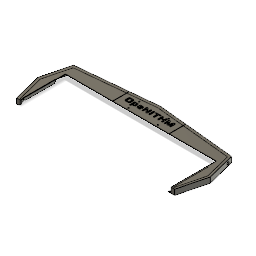
Frame v10 (Autodesk Fusion 360 design; units mm, degrees)
Autodesk Fusion 360 part; units mm, degrees
sketch "Sketch1" plane through (0, 0, 0) normal (0, 1, 0) x (1, 0, 0)
  line L0 (240, 0) -> (240, -144)
  line L1 (240, -144) -> (252, -144)
  line L2 (252, -144) -> (275, -53)
  line L3 (275, -53) -> (252, 38)
  line L4 (252, 38) -> (0, 63)
  line L5 (0, 63) -> (0, 0)
  line L6 (0, 0) -> (240, 0)
  dimension "d1" = 63
  dimension "d2" = 12
  dimension "d4" = 240
  dimension "d5" = 144
  dimension "d6" = 35
  dimension "d7" = 12
  dimension "d8" = 182
  measures "d1" distance of L5.end
extrude "Extrude1" add sketch "Sketch1" along normal blind 17.5 makes body 1
sketch "Sketch2" plane through (0, 0, 0) normal (0, -1, 0) x (1, 0, 0)
  line L0 (240, 0) -> (0, 0)
  line L1 (0, 0) -> (0, -63)
  line L2 (0, -63) -> (252, -38)
  line L3 (252, -38) -> (275, 53)
  line L4 (275, 53) -> (252, 144)
  line L5 (252, 144) -> (240, 144)
  line L6 (240, 144) -> (240, 0)
  line L7 (0, -55) -> (245.8682, -30.6083)
  line L8 (245.8682, -30.6083) -> (267, 53)
  line L9 (0, -55) -> (0, 0)
  line L10 (240, 0) -> (0, 0)
  line L11 (240, 0) -> (240, 139)
  line L12 (275, 53) -> (267, 53) construction
  line L13 (0, -63) -> (0, -55) construction
  line L14 (240, 139) -> (245.2637, 139)
  line L15 (245.2637, 139) -> (267, 53)
  dimension "d11" = 5
  dimension "d12" = 8
  dimension "d13" = 8
extrude "Extrude2" cut sketch "Sketch2" against normal blind 16 contours L0 L1 L6 L7 L8 L9 L10 L11 L14 L15 bodies 1
sketch "Sketch3" plane through (0, 0, 0) normal (-1, 0, 0) x (0, 0, 1)
  line L0 (-55, 0) -> (-55, 16)
  line L1 (-55, 16) -> (0, 16)
  line L2 (0, 16) -> (0, 17.5)
  line L3 (0, 17.5) -> (-63, 17.5)
  line L4 (-63, 17.5) -> (-63, 0)
  line L5 (-63, 0) -> (-55, 0)
  circle A0 centre (-22.6083, 8) radius 4
  line L6 (53, 0) -> (-30.6083, 0)
  line L7 (-30.6083, 0) -> (-30.6083, 16)
  dimension "d16" = 8
  dimension "d17" = 8
  dimension "d18" = 8
  measures "d16" diameter of A0
  measures "d17" distance of L6
  measures "d18" distance of L7
extrude "Extrude3" cut sketch "Sketch3" against normal through all contours A0 bodies 1
sketch "Sketch4" plane through (0, 0, 0) normal (0, 0, 1) x (1, 0, 0)
  line L0 (0, 16) -> (240, 16)
  line L1 (240, 16) -> (240, 17.5)
  line L2 (240, 17.5) -> (0, 17.5)
  line L3 (0, 17.5) -> (0, 16)
  line L4 (-8, 4) -> (8, 4)
  arc A0 (8, 4) -> (8, 12) centre (8, 8) ccw
  line L5 (8, 12) -> (-8, 12)
  arc A1 (-8, 12) -> (-8, 4) centre (-8, 8) ccw
  line L6 (-8, 8) -> (8, 8) construction
  line L7 (0, 0) -> (0, 17.5)
  line L8 (245.8682, 0) -> (0, 0)
  dimension "d20" = 8
  dimension "d21" = 12
  dimension "d22" = 8
  measures "d20" distance of L4 L5
  measures "d22" distance of L6 L8
extrude "Extrude4" cut sketch "Sketch4" against normal through all contours L4 A0 L5 L7 bodies 1
mirror "Mirror1" about plane through (0, 0, 0) normal (1, 0, 0) of "Extrude1", "Extrude2", "Extrude3", "Extrude4" makes body 2
combine "Combine1" operation add target body 1 tool bodies 2
sketch "Sketch5" plane through (0, 0, 144) normal (0, 0, 1) x (1, 0, 0)
  line L0 (240, 0) -> (252, 0)
  line L1 (252, 0) -> (252, 17.5)
  line L2 (252, 17.5) -> (240, 17.5)
  line L3 (240, 17.5) -> (240, 0)
  line L4 (245.8682, 0) -> (0, 0)
  line L5 (240, 0) -> (230, 0)
  line L6 (240, 3.7) -> (230, 0)
  line L7 (240, 0) -> (240, 3.7)
  dimension "d25" = 10
  dimension "d26" = 3.7
  measures "d26" distance of L4.end
extrude "Extrude5" add sketch "Sketch5" against normal blind 5 contours L3 L4 L5 L6 L7 bodies 1
sketch "Sketch6" plane through (0, 0, 144) normal (0, 0, 1) x (1, 0, 0)
  line L0 (-252, 0) -> (-240, 0)
  line L1 (-240, 0) -> (-240, 17.5)
  line L2 (-240, 17.5) -> (-252, 17.5)
  line L3 (-252, 17.5) -> (-252, 0)
  line L4 (-240, 0) -> (-240, 3.7)
  line L5 (-250, 0) -> (-240, 3.7)
  line L6 (-240, 0) -> (-250, 0)
  dimension "d29" = 3.7
  dimension "d30" = 10
  measures "d29" distance of origin
extrude "Extrude6" cut sketch "Sketch6" against normal blind 5 contours L0 L1 L4 L5 L6 bodies 1
ref_plane "WorkPlane1" through (0, 22.5, 40.5) normal (0, 1, 0) x (0, 0, 1)
sketch "Sketch7" plane through (0, 22.5, 0) normal (0, 1, 0) x (-1, 0, 0)
  line L0 (0, -41.653) -> (0, -63) construction
  line L1 (73.6847, -25.1213) -> (73.6847, -34.9739)
  spline S0 degree 2 poles (73.6847, -34.9739) (73.6847, -37.7889) (70.166, -37.7889) knots 0 0 0 1 1 1
  line L2 (70.166, -37.7889) -> (61.7209, -37.7889)
  spline S1 degree 2 poles (61.7209, -37.7889) (58.2021, -37.7889) (58.2021, -34.9739) knots 0 0 0 1 1 1
  line L3 (58.2021, -34.9739) -> (58.2021, -25.1213)
  spline S2 degree 2 poles (58.2021, -25.1213) (58.2021, -22.3062) (61.7209, -22.3062) knots 0 0 0 1 1 1
  line L4 (61.7209, -22.3062) -> (70.166, -22.3062)
  spline S3 degree 2 poles (70.166, -22.3062) (73.6847, -22.3062) (73.6847, -25.1213) knots 0 0 0 1 1 1
  spline S4 degree 2 poles (70.4005, -25.0509) (70.4005, -24.3002) (69.4622, -24.3002) knots 0 0 0 1 1 1
  line L5 (69.4622, -24.3002) -> (62.4246, -24.3002)
  spline S5 degree 2 poles (62.4246, -24.3002) (61.4863, -24.3002) (61.4863, -25.0509) knots 0 0 0 1 1 1
  line L6 (61.4863, -25.0509) -> (61.4863, -35.0443)
  spline S6 degree 2 poles (61.4863, -35.0443) (61.4863, -35.7949) (62.4246, -35.7949) knots 0 0 0 1 1 1
  line L7 (62.4246, -35.7949) -> (69.4622, -35.7949)
  spline S7 degree 2 poles (69.4622, -35.7949) (70.4005, -35.7949) (70.4005, -35.0443) knots 0 0 0 1 1 1
  line L8 (70.4005, -35.0443) -> (70.4005, -25.0509)
  line L9 (52.8552, -17.3799) -> (52.8552, -33.5664)
  line L10 (52.8552, -33.5664) -> (43.7063, -33.5664)
  spline S8 degree 2 poles (43.7063, -33.5664) (40.4221, -33.5664) (40.4221, -30.939) knots 0 0 0 1 1 1
  line L11 (40.4221, -30.939) -> (40.4221, -24.9336)
  spline S9 degree 2 poles (40.4221, -24.9336) (40.4221, -22.3062) (43.7063, -22.3062) knots 0 0 0 1 1 1
  line L12 (43.7063, -22.3062) -> (49.8056, -22.3062)
  line L13 (49.8056, -22.3062) -> (49.8056, -17.3799)
  line L14 (49.8056, -17.3799) -> (52.8552, -17.3799)
  line L15 (49.8056, -24.0656) -> (44.2928, -24.0656)
  spline S10 degree 2 poles (44.2928, -24.0656) (43.4718, -24.0656) (43.4718, -24.7225) knots 0 0 0 1 1 1
  line L16 (43.4718, -24.7225) -> (43.4718, -31.1501)
  spline S11 degree 2 poles (43.4718, -31.1501) (43.4718, -31.8069) (44.2928, -31.8069) knots 0 0 0 1 1 1
  line L17 (44.2928, -31.8069) -> (49.8056, -31.8069)
  line L18 (49.8056, -31.8069) -> (49.8056, -24.0656)
  line L19 (35.319, -24.9336) -> (35.319, -30.939)
  spline S12 degree 2 poles (35.319, -30.939) (35.319, -33.5664) (32.0348, -33.5664) knots 0 0 0 1 1 1
  line L20 (32.0348, -33.5664) -> (26.6393, -33.5664)
  spline S13 degree 2 poles (26.6393, -33.5664) (23.3551, -33.5664) (23.3551, -30.939) knots 0 0 0 1 1 1
  line L21 (23.3551, -30.939) -> (23.3551, -27.3498)
  line L22 (23.3551, -27.3498) -> (32.2694, -27.3498)
  line L23 (32.2694, -27.3498) -> (32.2694, -24.7225)
  spline S14 degree 2 poles (32.2694, -24.7225) (32.2694, -24.0656) (31.4483, -24.0656) knots 0 0 0 1 1 1
  line L24 (31.4483, -24.0656) -> (23.8243, -24.0656)
  line L25 (23.8243, -24.0656) -> (23.8243, -22.3062)
  line L26 (23.8243, -22.3062) -> (32.0348, -22.3062)
  spline S15 degree 2 poles (32.0348, -22.3062) (35.319, -22.3062) (35.319, -24.9336) knots 0 0 0 1 1 1
  line L27 (32.2694, -29.1092) -> (26.4047, -29.1092)
  line L28 (26.4047, -29.1092) -> (26.4047, -31.1501)
  spline S16 degree 2 poles (26.4047, -31.1501) (26.4047, -31.807) (27.2258, -31.807) knots 0 0 0 1 1 1
  line L29 (27.2258, -31.807) -> (31.4483, -31.807)
  spline S17 degree 2 poles (31.4483, -31.807) (32.2694, -31.807) (32.2694, -31.1501) knots 0 0 0 1 1 1
  line L30 (32.2694, -31.1501) -> (32.2694, -29.1092)
  line L31 (18.0064, -22.3062) -> (18.0064, -37.7889)
  line L32 (18.0064, -37.7889) -> (14.253, -37.7889)
  line L33 (14.253, -37.7889) -> (5.5733, -26.3411)
  line L34 (5.5733, -26.3411) -> (5.5733, -37.7889)
  line L35 (5.5733, -37.7889) -> (2.2891, -37.7889)
  line L36 (2.2891, -37.7889) -> (2.2891, -22.3062)
  line L37 (2.2891, -22.3062) -> (6.0425, -22.3062)
  line L38 (6.0425, -22.3062) -> (14.7222, -33.754)
  line L39 (14.7222, -33.754) -> (14.7222, -22.3062)
  line L40 (14.7222, -22.3062) -> (18.0064, -22.3062)
  line L41 (-3.2868, -22.3062) -> (-3.2868, -37.7889)
  line L42 (-3.2868, -37.7889) -> (-6.571, -37.7889)
  line L43 (-6.571, -37.7889) -> (-6.571, -22.3062)
  line L44 (-6.571, -22.3062) -> (-3.2868, -22.3062)
  line L45 (-10.9448, -35.7949) -> (-10.9448, -37.7889)
  line L46 (-10.9448, -37.7889) -> (-27.3658, -37.7889)
  line L47 (-27.3658, -37.7889) -> (-27.3658, -35.7949)
  line L48 (-27.3658, -35.7949) -> (-20.7974, -35.7949)
  line L49 (-20.7974, -35.7949) -> (-20.7974, -22.3062)
  line L50 (-20.7974, -22.3062) -> (-17.5132, -22.3062)
  line L51 (-17.5132, -22.3062) -> (-17.5132, -35.7949)
  line L52 (-17.5132, -35.7949) -> (-10.9448, -35.7949)
  line L53 (-31.7615, -22.3062) -> (-31.7615, -37.7889)
  line L54 (-31.7615, -37.7889) -> (-35.0457, -37.7889)
  line L55 (-35.0457, -37.7889) -> (-35.0457, -31.5724)
  line L56 (-35.0457, -31.5724) -> (-43.96, -31.5724)
  line L57 (-43.96, -31.5724) -> (-43.96, -37.7889)
  line L58 (-43.96, -37.7889) -> (-47.2442, -37.7889)
  line L59 (-47.2442, -37.7889) -> (-47.2442, -22.3062)
  line L60 (-47.2442, -22.3062) -> (-43.96, -22.3062)
  line L61 (-43.96, -22.3062) -> (-43.96, -29.5784)
  line L62 (-43.96, -29.5784) -> (-35.0457, -29.5784)
  line L63 (-35.0457, -29.5784) -> (-35.0457, -22.3062)
  line L64 (-35.0457, -22.3062) -> (-31.7615, -22.3062)
  line L65 (-52.8256, -22.3062) -> (-52.8256, -37.7889)
  line L66 (-52.8256, -37.7889) -> (-57.0482, -37.7889)
  line L67 (-57.0482, -37.7889) -> (-62.9128, -25.4966)
  line L68 (-62.9128, -25.4966) -> (-68.7775, -37.7889)
  line L69 (-68.7775, -37.7889) -> (-73.0001, -37.7889)
  line L70 (-73.0001, -37.7889) -> (-73.0001, -22.3062)
  line L71 (-73.0001, -22.3062) -> (-69.7158, -22.3062)
  line L72 (-69.7158, -22.3062) -> (-69.7158, -33.1206)
  line L73 (-69.7158, -33.1206) -> (-64.555, -22.3062)
  line L74 (-64.555, -22.3062) -> (-61.2708, -22.3062)
  line L75 (-61.2708, -22.3062) -> (-56.1099, -33.1206)
  line L76 (-56.1099, -33.1206) -> (-56.1099, -22.3062)
  line L77 (-56.1099, -22.3062) -> (-52.8256, -22.3062)
split_face "SplitFace1" 1 faces at (0, 17.5, -21) by curves path "Sketch7" along L7 S7 L8 S4 L5 S5 L6 S6 on bodies 1
split_face "SplitFace2" 1 faces at (59.5046, 17.5, -29.3503) by curves path "Sketch7" along S2 L4 S3 L1 S0 L2 S1 L3 on bodies 1
split_face "SplitFace3" 1 faces at (60.2506, 17.5, -28.6294) by curves path "Sketch7" along L15 S10 L16 S11 L17 L18 on bodies 1
split_face "SplitFace4" 1 faces at (65.5094, 17.5, -29.2408) by curves path "Sketch7" along L30 L27 L28 S16 L29 S17 on bodies 1
split_face "SplitFace5" 1 faces at (164, 17.5, -33.6667) by curves path "Sketch7" along S9 L12 L13 L14 L9 L10 S8 L11 on bodies 1
split_face "SplitFace6" 1 faces at (164, 17.5, -33.6667) by curves path "Sketch7" along S14 L24 L25 L26 S15 L19 S12 L20 S13 L21 L22 L23 on bodies 1
split_face "SplitFace7" 1 faces at (72.0586, 17.5, -28.4354) by curves path "Sketch7" along L35 L36 L37 L38 L39 L40 L31 L32 L33 L34 on bodies 1
split_face "SplitFace8" 1 faces at (164, 17.5, -33.6667) by curves path "Sketch7" along L41 L42 L43 L44 on bodies 1
split_face "SplitFace9" 1 faces at (166.1903, 17.5, -25.263) by curves path "Sketch7" along L48 L49 L50 L51 L52 L45 L46 L47 on bodies 1
split_face "SplitFace10" 1 faces at (173.1219, 17.5, -25.263) by curves path "Sketch7" along L58 L59 L60 L61 L62 L63 L64 L53 L54 L55 L56 L57 on bodies 1
split_face "SplitFace11" 1 faces at (179.7481, 17.5, -25.263) by curves path "Sketch7" along L69 L70 L71 L72 L73 L74 L75 L76 L77 L65 L66 L67 L68 on bodies 1
move_face "OffsetFaces1" offset -0.5 8 faces at (-60.3915, 17.5, -31.6897) (-51.8387, 17.5, -25.004) (-34.3025, 17.5, -27.7408) (-16.9117, 17.5, -31.283) (4.3816, 17.5, -32.628) (19.7026, 17.5, -31.2987) (32.8562, 17.5, -29.8912) (53.9204, 17.5, -31.0719) on bodies 1
sketch "Sketch8" plane through (0, 16, 0) normal (0, -1, 0) x (1, 0, 0)
  line L0 (0, -55) -> (245.8682, -30.6083)
  line L1 (245.8682, -30.6083) -> (267, 53)
  line L2 (240, 139) -> (240, 0)
  line L3 (240, 0) -> (-240, 0)
  line L4 (-240, 0) -> (-240, 139)
  line L5 (-267, 53) -> (-245.8682, -30.6083)
  line L6 (-245.8682, -30.6083) -> (0, -55)
  line L7 (75, -3.4651) -> (-75, -3.4651)
  line L8 (-75, -3.4651) -> (-75, -43.4651)
  line L9 (-75, -43.4651) -> (75, -43.4651)
  line L10 (75, -43.4651) -> (75, -3.4651)
  line L11 (75, -3.4651) -> (-75, -43.4651) construction
  line L12 (-75, -3.4651) -> (75, -43.4651) construction
  line L13 (-240, 139) -> (-245.2637, 139)
  line L14 (-245.2637, 139) -> (-267, 53)
  line L15 (267, 53) -> (245.2637, 139)
  line L16 (245.2637, 139) -> (240, 139)
  dimension "d37" = 150
  dimension "d38" = 40
  measures "d38" distance of origin
sketch "Sketch9" plane through (240, 0, 0) normal (-1, 0, 0) x (0, 0, 1)
  line L0 (139, 3.7) -> (144, 3.7)
  line L1 (144, 3.7) -> (144, 17.5)
  line L2 (144, 17.5) -> (0, 17.5)
  line L3 (0, 17.5) -> (0, 16)
  line L4 (0, 16) -> (139, 16)
  line L5 (0, 16) -> (29, 16)
  line L6 (29, 16) -> (36, 8)
  line L7 (36, 8) -> (128, 8)
  line L8 (128, 8) -> (135, 16)
  line L9 (139, 16) -> (139, 3.7)
  dimension "d41" = 29
  dimension "d43" = 7
  dimension "d44" = 8
  dimension "d45" = 9
  dimension "d46" = 7
extrude "Extrude8" add sketch "Sketch9" against normal blind 3 contours L4 L6 L7 L8 bodies 1
mirror "Mirror2" about plane through (0, 0, 0) normal (1, 0, 0) of "Extrude8"
ref_plane "WorkPlane2" through (90, 0, 0) normal (1, 0, 0) x (0, 1, 0)
split "Split1" by plane through (90, 0, 0) normal (1, 0, 0) bodies 1 makes body 3 at (140, 17.5, -18.0238)
ref_plane "WorkPlane3" through (-90, 0, 0) normal (1, 0, 0) x (0, 1, 0)
split "Split2" by plane through (-90, 0, 0) normal (1, 0, 0) bodies 1 makes body 4 at (-0.763, 17.5, -7.4354)
sketch "Sketch10" plane through (0, 16, 0) normal (0, -1, 0) x (1, 0, 0)
  line L0 (-90, 0) -> (-90, -46.0714)
  line L1 (-90, -46.0714) -> (0, -55)
  line L2 (0, -55) -> (90, -46.0714)
  line L3 (90, -46.0714) -> (90, 0)
  line L4 (90, 0) -> (-90, 0)
  line L5 (-46.99, -8.0241) -> (46.99, -8.0241) construction
  line L6 (46.99, -8.0241) -> (46.99, -42.3141) construction
  line L7 (46.99, -42.3141) -> (-46.99, -42.3141) construction
  line L8 (-46.99, -42.3141) -> (-46.99, -8.0241) construction
  line L9 (0, -42.3141) -> (0, -55) construction
  line L10 (-46.99, -8.0241) -> (-46.99, 0) construction
  line L11 (-46.99, -42.3141) -> (-46.99, -50.3383) construction
  circle A0 centre (-46.99, -8.0241) radius 2.15
  circle A1 centre (46.99, -8.0241) radius 2.15
  circle A2 centre (46.99, -42.3141) radius 2.15
  circle A3 centre (-46.99, -42.3141) radius 2.15
  dimension "d50" = 93.98
  dimension "d51" = 34.29
  dimension "d52" = 4.3
  measures "d51" distance of origin
  measures "d52" diameter of A1
extrude "Extrude9" add sketch "Sketch10" along normal blind 3 contours A0 | A1 | A2 | A3 bodies 4
sketch "Sketch11" plane through (0, 13, 0) normal (0, -1, 0) x (1, 0, 0)
  circle A0 centre (46.99, -42.3141) radius 2.15
  circle A1 centre (46.99, -42.3141) radius 2.15
  circle A2 centre (46.99, -8.0241) radius 2.15
  circle A3 centre (-46.99, -42.3141) radius 2.15
  circle A4 centre (-46.99, -8.0241) radius 2.15
hole "Hole1" at (46.99, 13, -42.3141) at (46.99, 13, -8.0241) at (-46.99, 13, -42.3141) at (-46.99, 13, -8.0241) direction (0, 1, 0) diameter 1.623 depth 3 tip angle 118 bodies 4
thread "Thread1" "ISO Metric profile 2.0 M2x0.4 6H"
equation "d39 = ( 180 / 2 ) * 1 mm"
equation "d40 = ( -180 / 2 ) * 1 mm"
named bodies: "Left Frame", "Right Frame", "Center Frame"
